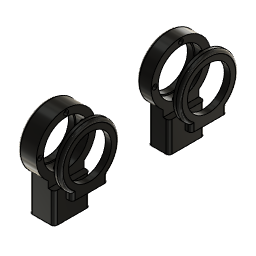
Lens Mounts (Autodesk Fusion 360 design; units mm, degrees)
Autodesk Fusion 360 part; units mm, degrees
sketch "Sketch1" plane through (0, 0, 0) normal (1, 0, 0) x (0, 1, 0)
  line L0 (0, 0) -> (-10, 0)
  line L1 (0, 0) -> (10, 0)
  line L2 (0, 0) -> (0, 51.1) construction
  circle A0 centre (0, 51.1) radius 19.125
  circle A1 centre (0, 51.1) radius 25
  line L3 (-10, 0) -> (-15, 0)
  line L4 (10, 0) -> (15, 0)
  line L5 (-15, 0) -> (-15, 31.1)
  line L6 (15, 0) -> (15, 31.1)
  dimension "d1" = 10
  dimension "d2" = 10
  dimension "d3" = 51.1
  dimension "d4" = 38.25
  dimension "d5" = 50
  dimension "d6" = 5
  dimension "d7" = 5
  constraint coincident L0.start L1.start
  constraint horizontal L0
  constraint parallel L0 L1
  constraint perpendicular L1 L2
  constraint coincident L2.end A0.centre
  constraint concentric A0 A1
  constraint parallel L0 L3
  constraint perpendicular L2 L4
  constraint coincident A1 L5.end
  constraint perpendicular L3 L5
  constraint coincident A1 L6.end
  constraint perpendicular L4 L6
  measures "d1" distance of L0.start L0.end
  measures "d2" distance of L0.start L1.end
  measures "d3" distance of L0.start L2.end
  measures "d4" diameter of A0
  measures "d5" diameter of A1
  measures "d6" distance of L0.end L3.end
  measures "d7" distance of L1.end L4.end
extrude "Extrude1" add sketch "Sketch1" along normal mid plane 15 makes body 1
ref_plane "WorkPlane1" through (-1.9957, 0, 76.1) normal (0, 0, 1) x (0, 1, 0)
sketch "Sketch2" plane through (-1.856, 0, 76.1) normal (0, 0, 1) x (1, 0, 0)
  line L0 (9.356, -25) -> (9.356, 25)
  line L1 (-5.644, 25) -> (-5.644, -25)
  line L2 (9.356, 0) -> (-5.644, 0) construction
  circle A0 centre (1.856, 0) radius 5
  dimension "d11" = 10
  constraint midpoint L0 L2.start
  constraint midpoint L1 L2.end
  constraint midpoint L2 A0.centre
  measures "d11" diameter of A0
sketch "Sketch3" plane through (-7.5, 0, 0) normal (-1, 0, 0) x (0, -1, 0)
  line L0 (-15, 0) -> (15, 0)
  circle A0 centre (0, 51.1) radius 19.125
  circle A1 centre (0, 51.1) radius 18
  line L1 (0, 69.1) -> (0, 70.225) construction
  line L2 (0, 69.1) -> (-6.4626, 69.1) construction
  line L3 (0, 69.1) -> (6.4626, 69.1) construction
  line L4 (-6.4626, 69.1) -> (0, 51.1) construction
  line L5 (0, 51.1) -> (6.4626, 69.1) construction
  line L6 (6.4626, 69.1) -> (6.0825, 68.0412)
  line L7 (-6.4626, 69.1) -> (-6.0825, 68.0412)
  line L8 (15, 0) -> (15, 31.1)
  arc A2 (15, 31.1) -> (-15, 31.1) centre (0, 51.1) ccw
  line L9 (-15, 31.1) -> (-15, 0)
  dimension "d16" = 36
  constraint coincident A1 L1.start
  constraint coincident A0 L1.end
  constraint vertical L1
  constraint coincident A0 L2.end
  constraint tangent A1 L2
  constraint perpendicular L1 L2
  constraint coincident A0 L3.end
  constraint tangent A1 L3
  constraint coincident A0.centre A1.centre
  constraint coincident A1 L6.end
  constraint coincident L5 L6.end
  constraint coincident L4 L7.end
  constraint coincident A1 L7.end
  measures "d16" diameter of A1
extrude "Extrude3" add sketch "Sketch3" against normal blind 5 contours A0 A1 L6 L7 picked at (-17.8528, 56.6831) bodies 1
sketch "Sketch4" plane through (0, 0, 0) normal (0, 0, -1) x (1, 0, 0)
  line L0 (7.5, -15) -> (7.5, 15)
  line L1 (7.5, 15) -> (-7.5, 15)
  line L2 (-7.5, 15) -> (-7.5, -15)
  line L3 (-7.5, -15) -> (7.5, -15)
  circle A0 centre (0, 0) radius 5.125
  dimension "d19" = 10.25
  constraint coincident A0.centre origin
  measures "d19" diameter of A0
extrude "Extrude4" cut sketch "Sketch4" against normal blind 10 contours A0 bodies 1
fillet "Fillet2" radius 2.5 3 edges at (-7.5, 0, 76.1) (-7.5, -15, 15.55) (-7.5, 15, 15.55) on bodies 1
sketch "Sketch5" plane through (7.5, 0, 0) normal (1, 0, 0) x (0, 1, 0)
  circle A0 centre (0, 51.1) radius 19.125
  line L0 (-15, 0) -> (15, 0)
  line L1 (15, 0) -> (15, 31.1)
  arc A1 (15, 31.1) -> (-15, 31.1) centre (0, 51.1) ccw
  line L2 (-15, 31.1) -> (-15, 0)
  line L3 (0, 70.225) -> (0, 73.1) construction
  circle A2 centre (0, 51.1) radius 22 construction
  line L4 (0, 51.1) -> (-22, 51.1) construction
  line L5 (0, 51.1) -> (0, 29.1) construction
  line L6 (0, 51.1) -> (22, 51.1) construction
  circle A3 centre (0, 73.1) radius 2
  circle A4 centre (22, 51.1) radius 2
  circle A5 centre (0, 29.1) radius 2
  circle A6 centre (-22, 51.1) radius 2
  dimension "d24" = 2.875
  dimension "d25" = 4
  dimension "d26" = 4
  dimension "d27" = 4
  dimension "d28" = 4
  constraint coincident A0 L3.start
  constraint vertical L3
  constraint concentric A0 A2
  constraint coincident L3.end A2
  constraint coincident A0.centre A1.centre
  constraint coincident A2 L4.end
  constraint horizontal L4
  constraint coincident A2 L5.end
  constraint perpendicular L4 L5
  constraint coincident A2 L6.end
  constraint parallel L4 L6
  constraint coincident L3.end A3.centre
  constraint coincident L6.end A4.centre
  constraint coincident L5.end A5.centre
  constraint coincident L4.end A6.centre
  measures "d24" distance of L3.start L3.end
  measures "d25" diameter of A3
  measures "d26" diameter of A4
  measures "d27" diameter of A5
  measures "d28" diameter of A6
extrude "Extrude5" cut sketch "Sketch5" against normal blind 2.5 contours A3 | A4 | A5 | A6 bodies 1
sketch "Sketch6" plane through (7.5, 0, 0) normal (1, 0, 0) x (0, 1, 0)
  circle A0 centre (22, 51.1) radius 2
  circle A1 centre (0, 29.1) radius 2
  circle A2 centre (0, 73.1) radius 2
  circle A3 centre (-22, 51.1) radius 2
  circle A4 centre (0, 51.1) radius 19.125
  line L0 (-15, 0) -> (15, 0)
  line L1 (15, 0) -> (15, 31.1)
  arc A5 (15, 31.1) -> (-15, 31.1) centre (0, 51.1) ccw
  line L2 (-15, 31.1) -> (-15, 0)
  line L3 (0, 25.475) -> (-15, 25.475)
  line L4 (0, 25.475) -> (15, 25.475)
  constraint coincident L2 L3.end
  constraint perpendicular L2 L3
  constraint coincident L1 L4.end
  constraint perpendicular L1 L4
extrude "Extrude6" add sketch "Sketch6" along normal blind 2.5 contours L0 L1 L2 L3 L4 bodies 1
extrude "Extrude7" add sketch "Sketch6" along normal blind 2.5 separate body contours A0 | A1 | A2 | A3 | L1 A5 L2 L3 L4 makes body 2
move_body "Move1" bodies 2 to x (1, 0, 0) y (0, 1, 0) z (0, 0, 1) at (15, 0, 0)
sketch "Sketch7" plane through (22.5, 0, 0) normal (-1, 0, 0) x (0, -1, 0)
  circle A0 centre (0, 51.1) radius 19.125
  line L0 (-15, 25.475) -> (15, 25.475)
  line L1 (15, 25.475) -> (15, 31.1)
  arc A1 (15, 31.1) -> (-15, 31.1) centre (0, 51.1) ccw
  line L2 (-15, 31.1) -> (-15, 25.475)
  line L3 (15, 25.475) -> (-15, 25.475)
  line L4 (-15, 25.475) -> (-15, 31.1)
  arc A2 (15, 31.1) -> (-15, 31.1) centre (0, 51.1) ccw
  line L5 (15, 31.1) -> (15, 25.475)
  circle A3 centre (-22, 51.1) radius 2
  circle A4 centre (0, 29.1) radius 2
  circle A5 centre (0, 73.1) radius 2
  circle A6 centre (22, 51.1) radius 2
  circle A7 centre (0, 51.1) radius 19.125
  circle A8 centre (22, 51.1) radius 1.75
  circle A9 centre (0, 73.1) radius 1.75
  circle A10 centre (-22, 51.1) radius 1.75
  circle A11 centre (0, 29.1) radius 1.75
  dimension "d36" = 3.5
  dimension "d37" = 3.5
  dimension "d38" = 3.5
  dimension "d39" = 3.5
  constraint concentric A6 A8
  constraint concentric A5 A9
  constraint concentric A3 A10
  constraint concentric A4 A11
  measures "d36" diameter of A8
  measures "d37" diameter of A9
  measures "d38" diameter of A10
  measures "d39" diameter of A11
extrude "Extrude8" add sketch "Sketch7" along normal blind 2 contours A8 | A9 | A10 | A11 bodies 2
extrude "Extrude9" add 1 faces at (10, -5, 8.4917) along direction (1, 0, 0) blind 2.5 on bodies 1 bodies 1
extrude "Extrude10" add 1 faces at (25, -0.4764, 27.6595) along direction (1, 0, 0) blind 2.5 on bodies 2 bodies 2
extrude "Extrude11" add 1 faces at (7.5, 7.9661, 29.0942) along direction (1, 0, 0) blind 1 on bodies 1 bodies 1
extrude "Extrude12" cut 1 faces at (22.5, -7.8865, 29.1187) along direction (1, 0, 0) blind 1 on bodies 2 bodies 2
extrude "Extrude13" add 1 faces at (12.5, -5, 8.4917) along direction (1, 0, 0) blind 1 on bodies 1 bodies 1
extrude "Extrude14" add 1 faces at (27.5, -0.4764, 27.6595) along direction (1, 0, 0) blind 1 on bodies 2 bodies 2
extrude "Extrude15" add 4 faces at (5, -0.1705, 29.6528) (5, -22.3112, 50.6198) (5, 0.5251, 74.0392) (5, 21.6888, 50.6198) along direction (1, 0, 0) blind 1 on bodies 1 bodies 1
extrude "Extrude16" cut 4 faces at (20.5, -22.1298, 50.5313) (20.5, 0.482, 72.5975) (20.5, 21.8702, 50.5313) (20.5, -0.699, 28.5674) along direction (1, 0, 0) blind 1 on bodies 2 bodies 2
copy_body "CopyPasteBodies1" bodies 2 1 makes body 3 makes body 4
move_body "Move2" bodies 3 4 to x (1, 0, 0) y (0, 1, 0) z (0, 0, 1) at (0, 100, 0)
extrude "Extrude17" cut 4 faces at (6, 121.6888, 50.6198) (6, 100.5251, 74.0392) (6, 77.6888, 50.6198) (6, 99.1455, 29.697) along direction (-1, 0, 0) blind 2 on bodies 4 bodies 4
extrude "Extrude18" cut 1 faces at (8.5, 107.9661, 29.0942) along direction (-1, 0, 0) blind 2 on bodies 4 bodies 4
extrude "Extrude19" cut 1 faces at (13.5, 95, 16.9833) along direction (-1, 0, 0) blind 2 on bodies 4 bodies 4
extrude "Extrude20" cut 1 faces at (6.5, 107.9661, 29.0942) along direction (-1, 0, 0) blind 1.5 on bodies 4 bodies 4
extrude "Extrude21" cut 4 faces at (4, 77.6888, 50.6198) (4, 100.5251, 74.0392) (4, 121.6888, 50.6198) (4, 99.1455, 29.697) along direction (-1, 0, 0) blind 1.5 on bodies 4 bodies 4
sketch "Sketch8" plane through (23.5, 0, 0) normal (-1, 0, 0) x (0, -1, 0)
  circle A0 centre (-122, 51.1) radius 1.75
  circle A1 centre (-100, 29.1) radius 1.75
  circle A2 centre (-100, 73.1) radius 1.75
  circle A3 centre (-78, 51.1) radius 1.75
  circle A4 centre (-100, 51.1) radius 19.125
  line L0 (-115, 25.475) -> (-85, 25.475)
  line L1 (-85, 25.475) -> (-85, 31.1)
  arc A5 (-85, 31.1) -> (-115, 31.1) centre (-100, 51.1) ccw
  line L2 (-115, 31.1) -> (-115, 25.475)
  circle A6 centre (-22, 51.1) radius 1.75
  circle A7 centre (0, 29.1) radius 1.75
  circle A8 centre (0, 73.1) radius 1.75
  circle A9 centre (22, 51.1) radius 1.75
  circle A10 centre (0, 51.1) radius 19.125
  line L3 (-15, 25.475) -> (15, 25.475)
  line L4 (15, 25.475) -> (15, 31.1)
  arc A11 (15, 31.1) -> (-15, 31.1) centre (0, 51.1) ccw
  line L5 (-15, 31.1) -> (-15, 25.475)
  circle A12 centre (-100, 51.1) radius 18
  circle A13 centre (0, 51.1) radius 18
  dimension "d72" = 36
  dimension "d73" = 36
  constraint concentric A4 A12
  constraint concentric A10 A13
  measures "d72" diameter of A12
  measures "d73" diameter of A13
extrude "Extrude22" add sketch "Sketch8" against normal blind 5 contours A4 | A10 bodies 2 3
extrude "Extrude23" cut 1 faces at (11.5, 95, 16.9833) along direction (-1, 0, 0) blind 1.5 on bodies 4 bodies 4
fillet "Fillet5" radius 2.5 10 edges at (13.5, 15, 12.7375) (13.5, -15, 12.7375) (28.5, 0, 76.1) (28.5, 15, 28.2875) (28.5, -15, 28.2875) (28.5, 100, 76.1) (28.5, 115, 28.2875) (28.5, 85, 28.2875) (10, 115, 12.7375) (10, 85, 12.7375) on bodies 1 2 3 4
equation "d24 = ( 5.750 / 2 ) * 1 mm"
